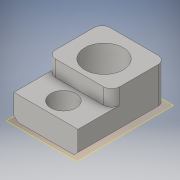
# Autodesk Inventor part: holder_test
Saved by Autodesk Inventor 2016 (Build 200138000, 138)
## iProperties
Created: 2018-07-05
Part Number: holder_test
Material: Generic
Document SubType Name: Modeling
Designer: tar
Density: 1 g/cm^3
Appearance: Default
Author: tar
Autodesk Inventor part; units mm, degrees
ref_plane "YZ Plane" through (0, 0, 0) normal (1, 0, 0) x (0, 1, 0)
ref_plane "XZ Plane" through (0, 0, 0) normal (0, 1, 0) x (-1, 0, 0)
sketch "Sketch1" plane through (0, 0, 0) normal (0, 0, 1) x (1, 0, 0)
  line L0 (0, 0) -> (8, 0)
  line L1 (8, 0) -> (8, 11)
  line L2 (8, 11) -> (0, 11)
  line L3 (0, 11) -> (0, 0)
  dimension "d0" = 8
  dimension "d1" = 11
  constraints: 8 end point, 2 parallel, 1 horizontal, 1 perpendicular
  measures "d0" distance of L1.end L2.end
  measures "d1" distance of L0.end L1.end
extrude "Extrusion1" add sketch "Sketch1" along normal blind 5
sketch "Sketch2" plane through (0, 0, 5) normal (0, 0, 1) x (1, 0, 0)
  circle A0 centre (4, 7.251) radius 2.4
  circle A1 centre (4, 2.176) radius 1.575
  line L0 (4, 10.5689) -> (4, 1.2689) construction
  line L1 (0, 11) -> (0, 0) projected
  line L2 (8, 0) -> (8, 11) projected
  dimension "d4" = 3.15
  dimension "d5" = 4.8
  dimension "d6" = 1.1
  dimension "d7" = 4
  dimension "d8" = 4
  constraints: 2 centre point, 2 end point, 2 point on line, 1 vertical
  measures "d4" diameter of A1
  measures "d5" diameter of A0
  measures "d7" distance between parallel lines of L1 L0
  measures "d8" distance between parallel lines of L2 L0
extrude "Extrusion2" cut sketch "Sketch2" against normal blind 7
sketch "Sketch4" plane through (0, 0, 5) normal (0, 0, 1) x (1, 0, 0)
  line L0 (0, 0) -> (8, 0)
  line L1 (8, 0) -> (8, 4.2)
  line L2 (8, 4.2) -> (0, 4.2)
  line L3 (0, 4.2) -> (0, 0)
  line L4 (8, 0) -> (8, 11) projected
  circle A0 centre (4, 7.251) radius 2.4 projected
  circle A1 centre (4, 2.176) radius 1.575 projected
  dimension "d14" = 4.2
  constraints: 8 end point, 2 parallel, 1 collinear, 1 horizontal, 1 perpendicular, 1 other
  measures "d14" distance between parallel lines of L0 L2
extrude "Extrusion4" cut sketch "Sketch4" against normal blind 2 contours L3 L2 L1 L0
fillet "Rundung1" radius 1 4 edges at (0, 11, 2.5) (8, 11, 2.5) (0, 4.2, 4) (8, 4.2, 4)
chamfer "Fase1" distance 0.5 angle 45 5 edges at (8, 5, 0) (7.7071, 10.7071, 0) (4, 11, 0) (0.2929, 10.7071, 0) (0, 5, 0)
body "Solid1"
